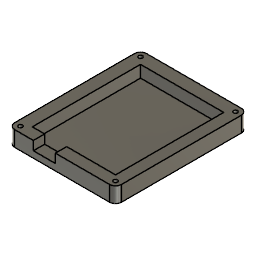
hackpad bottom (Autodesk Fusion 360 design; units mm, degrees)
part number: 2026-01-07-17-07-04-938
part number: 2026-01-07-17-11-01-476
Autodesk Fusion 360 part; units mm, degrees
sketch "Sketch1" plane through (0, 0, 0) normal (0, 0, 1) x (1, 0, 0) in component "chrif's perfect hackpad"
  line L0 (-37.215, 51.0468) -> (32.785, 51.0468)
  line L1 (32.785, 51.0468) -> (32.785, -39.9532)
  line L2 (32.785, -39.9532) -> (-37.215, -39.9532)
  line L3 (-37.215, -39.9532) -> (-37.215, 51.0468)
  line L4 (-47.715, 61.5468) -> (42.285, 61.5468)
  line L5 (42.285, 61.5468) -> (42.285, -49.4532)
  line L6 (42.285, -49.4532) -> (-47.715, -49.4532)
  line L7 (-47.715, -49.4532) -> (-47.715, 61.5468)
  circle A0 centre (-42.715, -44.4532) radius 1.7
  circle A1 centre (37.285, -44.4532) radius 1.7
  circle A2 centre (37.285, 56.5468) radius 1.7
  circle A3 centre (-42.715, 56.5468) radius 1.7
  circle A4 centre (-42.715, -44.4532) radius 3
  circle A5 centre (37.285, -44.4532) radius 3
  circle A6 centre (37.285, 56.5468) radius 3
  circle A7 centre (-42.715, 56.5468) radius 3
  dimension "d1" = 70
  dimension "d2" = 91
  dimension "d3" = 90
  dimension "d4" = 111
  dimension "d5" = 9.5
  dimension "d6" = 9.5
  dimension "d7" = 3.4
  dimension "d8" = 5
  dimension "d9" = 5
  dimension "d10" = 3.4
  dimension "d11" = 5
  dimension "d12" = 5
  dimension "d13" = 3.4
  dimension "d14" = 5
  dimension "d15" = 5
  dimension "d16" = 3.4
  dimension "d17" = 5
  dimension "d18" = 5
  dimension "d19" = 6
  dimension "d20" = 6
  dimension "d21" = 6
  dimension "d22" = 6
  constraint horizontal L0
  constraint vertical L1
  constraint horizontal L2
  constraint vertical L3
  constraint horizontal L4
  constraint vertical L5
  constraint horizontal L6
  constraint vertical L7
  constraint concentric A0 A4
  constraint concentric A1 A5
  constraint concentric A2 A6
  constraint concentric A3 A7
  measures "d1" distance of L1.end L2.end
  measures "d2" distance of L0.end L1.end
  measures "d3" distance of L5.end L6.end
  measures "d4" distance of L4.end L5.end
  measures "d5" distance of L2 L6
  measures "d6" distance of L1 L5
  measures "d7" diameter of A0
  measures "d8" distance of L7 A0.centre
  measures "d9" distance of L6 A0.centre
  measures "d10" diameter of A1
  measures "d11" distance of L5 A1.centre
  measures "d12" distance of L6 A1.centre
  measures "d13" diameter of A2
  measures "d14" distance of L4 A2.centre
  measures "d15" distance of L5 A2.centre
  measures "d16" diameter of A3
  measures "d17" distance of L4 A3.centre
  measures "d18" distance of L7 A3.centre
  measures "d19" diameter of A4
  measures "d20" diameter of A5
  measures "d21" diameter of A6
  measures "d22" diameter of A7
extrude "Extrude1" add sketch "Sketch1" along normal blind 9.9 from surface at 3.1 contours A4 | A5 | A6 | A7 makes body 1 at (-45.7113, 56.3972, 9.7) makes body 2 at (40.2812, -44.6028, 9.7) makes body 3 at (34.2887, 56.3972, 9.7) makes body 4 at (-45.7113, -44.6028, 9.7) in component "chrif's perfect hackpad"
extrude "Extrude2" add sketch "Sketch1" along normal blind 13 contours L4 L5 L6 L7 bodies 1 2 3 4 in component "chrif's perfect hackpad"
sketch "Sketch2" plane through (0, 0, 13) normal (0, 0, 1) x (-1, 0, 0) in component "chrif's perfect hackpad"
  circle A0 centre (42.715, -56.5468) radius 1.7
  circle A1 centre (42.715, 44.4532) radius 1.7
  line L0 (-32.785, 39.9532) -> (37.215, 39.9532)
  line L1 (37.215, 39.9532) -> (37.215, -51.0468)
  line L2 (37.215, -51.0468) -> (-32.785, -51.0468)
  line L3 (-32.785, -51.0468) -> (-32.785, 39.9532)
  line L4 (47.715, 49.4532) -> (-42.285, 49.4532)
  line L5 (-42.285, 49.4532) -> (-42.285, -61.5468)
  line L6 (-42.285, -61.5468) -> (47.715, -61.5468)
  line L7 (47.715, -61.5468) -> (47.715, 49.4532)
  circle A2 centre (-37.285, 44.4532) radius 1.7
  circle A3 centre (-37.285, -56.5468) radius 1.7
  line L8 (8.336, 49.4532) -> (26.836, 49.4532)
  line L9 (26.836, 49.4532) -> (26.836, 39.9532)
  line L10 (26.836, 39.9532) -> (8.336, 39.9532)
  line L11 (8.336, 39.9532) -> (8.336, 49.4532)
  line L12 (-42.285, -61.5468) -> (-42.285, 49.4532)
  dimension "d28" = 18.5
  dimension "d29" = 50.621
  constraint horizontal L8
  constraint vertical L9
  constraint horizontal L10
  constraint vertical L11
  constraint coincident L0 L9.end
  constraint coincident L4 L8.start
  measures "d28" distance of L9 L11
  measures "d29" distance of L11 L12
extrude "Extrude3" cut sketch "Sketch2" against normal blind 7.5 contours L0 L4 L8 L9 L10 L11 bodies 1 in component "chrif's perfect hackpad"
fillet "Fillet1" radius 5 1 edges at (42.285, 61.5468, 6.5) on bodies 1 in component "chrif's perfect hackpad"
fillet "Fillet2" radius 5 1 edges at (-47.715, 61.5468, 6.5) on bodies 1 in component "chrif's perfect hackpad"
fillet "Fillet3" radius 5 1 edges at (-47.715, -49.4532, 6.5) on bodies 1 in component "chrif's perfect hackpad"
fillet "Fillet4" radius 5 1 edges at (42.285, -49.4532, 6.5) on bodies 1 in component "chrif's perfect hackpad"
extrude "Extrude4" add sketch "Sketch1" along normal blind 3 contours L0 L1 L2 L3 bodies 1 in component "chrif's perfect hackpad"
sketch "Sketch3" plane through (0, 0, 0) normal (0, 0, -1) x (1, 0, 0) in component "chrif's perfect hackpad"
  arc A0 (42.285, 44.4532) -> (37.285, 49.4532) centre (37.285, 44.4532) ccw
  line L0 (37.285, 49.4532) -> (-42.715, 49.4532)
  arc A1 (-42.715, 49.4532) -> (-47.715, 44.4532) centre (-42.715, 44.4532) ccw
  line L1 (-47.715, 44.4532) -> (-47.715, -56.5468)
  arc A2 (-47.715, -56.5468) -> (-42.715, -61.5468) centre (-42.715, -56.5468) ccw
  line L2 (-42.715, -61.5468) -> (37.285, -61.5468)
  arc A3 (37.285, -61.5468) -> (42.285, -56.5468) centre (37.285, -56.5468) ccw
  line L3 (42.285, -56.5468) -> (42.285, 44.4532)
  circle A4 centre (37.285, 44.4532) radius 3
  circle A5 centre (-42.715, -56.5468) radius 3
  circle A6 centre (37.285, -56.5468) radius 3
  circle A7 centre (-42.715, 44.4532) radius 3
  line L4 (25.2067, 35.4447) -> (-9.5084, 35.4447) construction
  line L5 (-9.5084, 35.4447) -> (-9.5084, 24.6183) construction
  line L6 (-9.5084, 24.6183) -> (25.2067, 24.6183) construction
  line L7 (25.2067, 24.6183) -> (25.2067, 35.4447) construction
  dimension "d42" = 3
  text T0 "chrifs \nperfect\nhackpad" font "Arial" height 3 align left top in box 34.7151 x 10.8264 at (25.2067, 35.4447) x (-1, 0) y (0, -1) spacing 1
extrude "Extrude5" add sketch "Sketch3" along normal blind 0.2 text T0 bodies 1 in component "chrif's perfect hackpad"
component "chrif's perfect hackpad" placed x (1, 0, 0) y (0, 1, 0) z (0, 0, 1) at (0, 0, 0)
equation "d43 = 'chrifs  perfect hackpad'"
